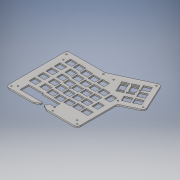
# Autodesk Inventor part: steelplate right
Saved by Autodesk Inventor 2016 (Build 200138000, 138)
## iProperties
Created: 2016-01-27
Part Number: steelplate right
Material: Generic
Document SubType Name: Sheet Metal
Designer: Fab Lab
Density: 1 g/cm^3
Sheet Metal Rule: Default
Appearance: Default
Author: Fab Lab
Autodesk Inventor part; units mm, degrees
ref_plane "YZ Plane" through (0, 0, 0) normal (1, 0, 0) x (0, 1, 0)
ref_plane "XZ Plane" through (0, 0, 0) normal (0, 1, 0) x (-1, 0, 0)
ref_plane "XY Plane" through (0, 0, 0) normal (0, 0, 1) x (1, 0, 0)
sketch "Sketch1" plane through (0, 0, 0) normal (0, 1, 0) x (-1, 0, 0)
  line L0 (-203.0862, 221.0628) -> (-258.5956, 221.0628)
  line L1 (-287.8818, 221.0628) -> (-350.173, 221.0628)
  line L2 (-342.06, 221.0628) -> (-350.173, 221.0628)
  line L3 (-277.102195, 211.948924) -> (-279.894095, 211.949068)
  line L4 (-269.4008, 215.9498) -> (-269.4008, 211.949)
  line L5 (-218.894185, 211.949) -> (-269.4008, 211.949)
  line L6 (-269.4008, 215.9498) -> (-267.9008, 215.9498)
  line L7 (-278.60199, 215.949801) -> (-277.10199, 215.949724)
  line L8 (-267.9008, 215.9498) -> (-258.5956, 221.0628)
  line L9 (-287.8818, 221.0628) -> (-278.5767, 215.9498)
  line L10 (-291.226534, 207.296649) -> (-279.894334, 207.296068)
  line L11 (-279.894095, 211.949068) -> (-279.894334, 207.296068)
  spline S0 degree 3 poles (-361.2149, 128.8298) (-358.7492, 129.9795) (-357.173, 132.4535) (-357.173, 135.174) knots 0 0 0 0 1 1 1 1
  line L12 (-361.2149, 128.8298) -> (-358.7492, 129.9795) construction
  line L13 (-358.7492, 129.9795) -> (-357.173, 132.4535) construction
  line L14 (-357.173, 132.4535) -> (-357.173, 135.174) construction
  spline S1 degree 3 poles (-280.219, 82.6328) (-281.241, 82.6328) (-282.2506, 82.409) (-283.1768, 81.9771) knots 0 0 0 0 1 1 1 1
  line L15 (-280.219, 82.6328) -> (-281.241, 82.6328) construction
  line L16 (-281.241, 82.6328) -> (-282.2506, 82.409) construction
  line L17 (-282.2506, 82.409) -> (-283.1768, 81.9771) construction
  line L18 (-357.172987, 214.0628) -> (-357.172987, 135.1741)
  line L19 (-196.0862, 89.6328) -> (-196.0862, 214.0628)
  line L20 (-398.011196, 103.949092) -> (-372.0468, 48.2678)
  line L21 (-362.7448, 44.8818) -> (-283.1768, 81.9771)
  line L22 (-280.219, 82.6328) -> (-203.0862, 82.6328)
  spline S2 degree 3 poles (-196.0862, 214.0628) (-196.0862, 215.9193) (-196.8237, 217.6997) (-198.1365, 219.0125) knots 0 0 0 0 1 1 1 1
  line L23 (-196.0862, 214.0628) -> (-196.0862, 215.9193) construction
  line L24 (-196.0862, 215.9193) -> (-196.8237, 217.6997) construction
  line L25 (-196.8237, 217.6997) -> (-198.1365, 219.0125) construction
  line L26 (-198.1365, 219.0125) -> (-198.1365, 219.0125) construction
  line L27 (-198.1365, 219.0125) -> (-199.4492, 220.3253) construction
  line L28 (-199.4492, 220.3253) -> (-201.2297, 221.0628) construction
  line L29 (-201.2297, 221.0628) -> (-203.0862, 221.0628) construction
  spline S3 degree 3 poles (-350.173, 221.0628) (-352.0295, 221.0628) (-353.81, 220.3253) (-355.1228, 219.0125) knots 0 0 0 0 1 1 1 1
  line L30 (-350.173, 221.0628) -> (-352.0295, 221.0628) construction
  line L31 (-352.0295, 221.0628) -> (-353.81, 220.3253) construction
  line L32 (-353.81, 220.3253) -> (-355.1228, 219.0125) construction
  line L33 (-355.1228, 219.0125) -> (-355.1228, 219.0125) construction
  line L34 (-355.1228, 219.0125) -> (-356.4355, 217.6997) construction
  line L35 (-356.4355, 217.6997) -> (-357.173, 215.9193) construction
  line L36 (-357.173, 215.9193) -> (-357.172987, 214.0628) construction
  line L37 (-361.2149, 128.8298) -> (-394.6251, 113.2517)
  spline S4 degree 3 poles (-203.0862, 82.6328) (-199.2202, 82.6328) (-196.0862, 85.7667) (-196.0862, 89.6327) knots 0 0 0 0 1 1 1 1
  line L38 (-203.0862, 82.6328) -> (-199.2202, 82.6328) construction
  line L39 (-199.2202, 82.6328) -> (-196.0862, 85.7667) construction
  line L40 (-196.0862, 85.7667) -> (-196.0862, 89.6327) construction
  spline S5 degree 3 poles (-372.0468, 48.2678) (-370.413, 44.7642) (-366.2485, 43.2483) (-362.7448, 44.8818) knots 0 0 0 0 1 1 1 1
  line L41 (-372.0468, 48.2678) -> (-370.413, 44.7642) construction
  line L42 (-370.413, 44.7642) -> (-366.2485, 43.2483) construction
  line L43 (-366.2485, 43.2483) -> (-362.7448, 44.8818) construction
  spline S6 degree 3 poles (-394.6251, 113.2517) (-396.3077, 112.4671) (-397.6098, 111.0463) (-398.2448, 109.3017) knots 0 0 0 0 1 1 1 1
  line L44 (-394.6251, 113.2517) -> (-396.3077, 112.4671) construction
  line L45 (-396.3077, 112.4671) -> (-397.6098, 111.0463) construction
  line L46 (-397.6098, 111.0463) -> (-398.2448, 109.3017) construction
  line L47 (-398.2448, 109.3017) -> (-398.2448, 109.3017) construction
  line L48 (-398.2448, 109.3017) -> (-398.8798, 107.5571) construction
  line L49 (-398.8798, 107.5571) -> (-398.7958, 105.6317) construction
  line L50 (-398.7958, 105.6317) -> (-398.011196, 103.949092) construction
  line L51 (-277.10199, 215.949724) -> (-277.102195, 211.948924)
  line L52 (-291.894992, 194.449787) -> (-291.894457, 206.045087)
  line L53 (-251.675985, 192.447826) -> (-218.895085, 192.446313)
  line L54 (-218.895085, 192.446313) -> (-218.894185, 211.949)
  line L55 (-251.675892, 194.447826) -> (-291.894992, 194.449683)
  line L56 (-251.675892, 194.447826) -> (-251.675985, 192.447826)
  line L57 (-227.2963, 171.6071) -> (-211.7963, 171.6071)
  line L58 (-211.7963, 171.6071) -> (-211.7963, 184.4071)
  line L59 (-211.7963, 184.4071) -> (-227.2963, 184.4071)
  line L60 (-227.2963, 184.4071) -> (-227.2963, 171.6071)
  line L61 (-251.0963, 171.6071) -> (-235.5963, 171.6071)
  line L62 (-235.5963, 171.6071) -> (-235.5963, 184.4071)
  line L63 (-235.5963, 184.4071) -> (-251.0963, 184.4071)
  line L64 (-251.0963, 184.4071) -> (-251.0963, 171.6071)
  line L65 (-227.2963, 152.5071) -> (-211.7963, 152.5071)
  line L66 (-211.7963, 152.5071) -> (-211.7963, 165.3071)
  line L67 (-211.7963, 165.3071) -> (-227.2963, 165.3071)
  line L68 (-227.2963, 165.3071) -> (-227.2963, 152.5071)
  line L69 (-251.0963, 152.5071) -> (-235.5963, 152.5071)
  line L70 (-235.5963, 152.5071) -> (-235.5963, 165.3071)
  line L71 (-235.5963, 165.3071) -> (-251.0963, 165.3071)
  line L72 (-251.0963, 165.3071) -> (-251.0963, 152.5071)
  line L73 (-227.2963, 133.5071) -> (-211.7963, 133.5071)
  line L74 (-211.7963, 133.5071) -> (-211.7963, 146.3071)
  line L75 (-211.7963, 146.3071) -> (-227.2963, 146.3071)
  line L76 (-227.2963, 146.3071) -> (-227.2963, 133.5071)
  line L77 (-251.0963, 133.5071) -> (-235.5963, 133.5071)
  line L78 (-235.5963, 133.5071) -> (-235.5963, 146.3071)
  line L79 (-235.5963, 146.3071) -> (-251.0963, 146.3071)
  line L80 (-251.0963, 146.3071) -> (-251.0963, 133.5071)
  line L81 (-227.2963, 114.5071) -> (-211.7963, 114.5071)
  line L82 (-211.7963, 114.5071) -> (-211.7963, 127.3071)
  line L83 (-211.7963, 127.3071) -> (-227.2963, 127.3071)
  line L84 (-227.2963, 127.3071) -> (-227.2963, 114.5071)
  line L85 (-251.0963, 114.5071) -> (-235.5963, 114.5071)
  line L86 (-235.5963, 114.5071) -> (-235.5963, 127.3071)
  line L87 (-235.5963, 127.3071) -> (-251.0963, 127.3071)
  line L88 (-251.0963, 127.3071) -> (-251.0963, 114.5071)
  line L89 (-270.0539, 174.7882) -> (-254.5539, 174.7882)
  line L90 (-254.5539, 174.7882) -> (-254.5539, 187.5882)
  line L91 (-254.5539, 187.5882) -> (-270.0539, 187.5882)
  line L92 (-270.0539, 187.5882) -> (-270.0539, 174.7882)
  line L93 (-270.0539, 155.6882) -> (-254.5539, 155.6882)
  line L94 (-254.5539, 155.6882) -> (-254.5539, 168.4882)
  line L95 (-254.5539, 168.4882) -> (-270.0539, 168.4882)
  line L96 (-270.0539, 168.4882) -> (-270.0539, 155.6882)
  line L97 (-270.0539, 136.6882) -> (-254.5539, 136.6882)
  line L98 (-254.5539, 136.6882) -> (-254.5539, 149.4882)
  line L99 (-254.5539, 149.4882) -> (-270.0539, 149.4882)
  line L100 (-270.0539, 149.4882) -> (-270.0539, 136.6882)
  line L101 (-270.0539, 117.6882) -> (-254.5539, 117.6882)
  line L102 (-254.5539, 117.6882) -> (-254.5539, 130.4882)
  line L103 (-254.5539, 130.4882) -> (-270.0539, 130.4882)
  line L104 (-270.0539, 130.4882) -> (-270.0539, 117.6882)
  line L105 (-270.0539, 98.5882) -> (-254.5539, 98.5882)
  line L106 (-254.5539, 98.5882) -> (-254.5539, 111.3882)
  line L107 (-254.5539, 111.3882) -> (-270.0539, 111.3882)
  line L108 (-270.0539, 111.3882) -> (-270.0539, 98.5882)
  line L109 (-289.1803, 176.3757) -> (-273.6803, 176.3757)
  line L110 (-273.6803, 176.3757) -> (-273.6803, 189.1757)
  line L111 (-273.6803, 189.1757) -> (-289.1803, 189.1757)
  line L112 (-289.1803, 189.1757) -> (-289.1803, 176.3757)
  line L113 (-289.1803, 157.2757) -> (-273.6803, 157.2757)
  line L114 (-273.6803, 157.2757) -> (-273.6803, 170.0757)
  line L115 (-273.6803, 170.0757) -> (-289.1803, 170.0757)
  line L116 (-289.1803, 170.0757) -> (-289.1803, 157.2757)
  line L117 (-289.1803, 138.2757) -> (-273.6803, 138.2757)
  line L118 (-273.6803, 138.2757) -> (-273.6803, 151.0757)
  line L119 (-273.6803, 151.0757) -> (-289.1803, 151.0757)
  line L120 (-289.1803, 151.0757) -> (-289.1803, 138.2757)
  line L121 (-289.1803, 119.2757) -> (-273.6803, 119.2757)
  line L122 (-273.6803, 119.2757) -> (-273.6803, 132.0757)
  line L123 (-273.6803, 132.0757) -> (-289.1803, 132.0757)
  line L124 (-289.1803, 132.0757) -> (-289.1803, 119.2757)
  line L125 (-289.1803, 100.1757) -> (-273.6803, 100.1757)
  line L126 (-273.6803, 100.1757) -> (-273.6803, 112.9757)
  line L127 (-273.6803, 112.9757) -> (-289.1803, 112.9757)
  line L128 (-289.1803, 112.9757) -> (-289.1803, 100.1757)
  line L129 (-308.1764, 174.8083) -> (-292.6764, 174.8083)
  line L130 (-292.6764, 174.8083) -> (-292.6764, 187.6083)
  line L131 (-292.6764, 187.6083) -> (-308.1764, 187.6083)
  line L132 (-308.1764, 187.6083) -> (-308.1764, 174.8083)
  line L133 (-308.1764, 155.7083) -> (-292.6764, 155.7083)
  line L134 (-292.6764, 155.7083) -> (-292.6764, 168.5083)
  line L135 (-292.6764, 168.5083) -> (-308.1764, 168.5083)
  line L136 (-308.1764, 168.5083) -> (-308.1764, 155.7083)
  line L137 (-308.1764, 136.7083) -> (-292.6764, 136.7083)
  line L138 (-292.6764, 136.7083) -> (-292.6764, 149.5083)
  line L139 (-292.6764, 149.5083) -> (-308.1764, 149.5083)
  line L140 (-308.1764, 149.5083) -> (-308.1764, 136.7083)
  line L141 (-308.1764, 117.7083) -> (-292.6764, 117.7083)
  line L142 (-292.6764, 117.7083) -> (-292.6764, 130.5083)
  line L143 (-292.6764, 130.5083) -> (-308.1764, 130.5083)
  line L144 (-308.1764, 130.5083) -> (-308.1764, 117.7083)
  line L145 (-308.1764, 98.6083) -> (-292.6764, 98.6083)
  line L146 (-292.6764, 98.6083) -> (-292.6764, 111.4083)
  line L147 (-292.6764, 111.4083) -> (-308.1764, 111.4083)
  line L148 (-308.1764, 111.4083) -> (-308.1764, 98.6083)
  line L149 (-327.2289, 173.5307) -> (-311.7289, 173.5307)
  line L150 (-311.7289, 173.5307) -> (-311.7289, 186.3307)
  line L151 (-311.7289, 186.3307) -> (-327.2289, 186.3307)
  line L152 (-327.2289, 186.3307) -> (-327.2289, 173.5307)
  line L153 (-327.2289, 154.4307) -> (-311.7289, 154.4307)
  line L154 (-311.7289, 154.4307) -> (-311.7289, 167.2307)
  line L155 (-311.7289, 167.2307) -> (-327.2289, 167.2307)
  line L156 (-327.2289, 167.2307) -> (-327.2289, 154.4307)
  line L157 (-327.2289, 135.4307) -> (-311.7289, 135.4307)
  line L158 (-311.7289, 135.4307) -> (-311.7289, 148.2307)
  line L159 (-311.7289, 148.2307) -> (-327.2289, 148.2307)
  line L160 (-327.2289, 148.2307) -> (-327.2289, 135.4307)
  line L161 (-327.2289, 116.4307) -> (-311.7289, 116.4307)
  line L162 (-311.7289, 116.4307) -> (-311.7289, 129.2307)
  line L163 (-311.7289, 129.2307) -> (-327.2289, 129.2307)
  line L164 (-327.2289, 129.2307) -> (-327.2289, 116.4307)
  line L165 (-346.3289, 173.5307) -> (-330.8289, 173.5307)
  line L166 (-330.8289, 173.5307) -> (-330.8289, 186.3307)
  line L167 (-330.8289, 186.3307) -> (-346.3289, 186.3307)
  line L168 (-346.3289, 186.3307) -> (-346.3289, 173.5307)
  line L169 (-251.0963, 95.4071) -> (-235.5963, 95.4071)
  line L170 (-235.5963, 95.4071) -> (-235.5963, 108.2071)
  line L171 (-235.5963, 108.2071) -> (-251.0963, 108.2071)
  line L172 (-251.0963, 108.2071) -> (-251.0963, 95.4071)
  line L173 (-231.9963, 95.4071) -> (-216.4963, 95.4071)
  line L174 (-216.4963, 95.4071) -> (-216.4963, 108.2071)
  line L175 (-216.4963, 108.2071) -> (-231.9963, 108.2071)
  line L176 (-231.9963, 108.2071) -> (-231.9963, 95.4071)
  line L177 (-332.7989, 147.8041) -> (-332.7989, 163.3041)
  line L178 (-332.7989, 163.3041) -> (-345.5989, 163.3041)
  line L179 (-345.5989, 163.3041) -> (-345.5989, 147.8041)
  line L180 (-345.5989, 147.8041) -> (-332.7989, 147.8041)
  line L181 (-332.7989, 119.2041) -> (-332.7989, 134.7041)
  line L182 (-332.7989, 134.7041) -> (-345.5989, 134.7041)
  line L183 (-345.5989, 134.7041) -> (-345.5989, 119.2041)
  line L184 (-345.5989, 119.2041) -> (-332.7989, 119.2041)
  line L185 (-354.9415, 118.8037) -> (-368.9892, 112.2531)
  line L186 (-368.9892, 112.2531) -> (-363.5797, 100.6523)
  line L187 (-363.5797, 100.6523) -> (-349.5319, 107.2029)
  line L188 (-349.5319, 107.2029) -> (-354.9415, 118.8037)
  line L189 (-372.2276, 110.778) -> (-386.2753, 104.2274)
  line L190 (-386.2753, 104.2274) -> (-380.8658, 92.6266)
  line L191 (-380.866146, 92.626439) -> (-366.81815, 99.17662)
  line L192 (-366.818, 99.1772) -> (-372.2276, 110.778)
  line L193 (-364.1137, 93.4918) -> (-378.1614, 86.9412)
  line L194 (-378.1614, 86.9412) -> (-372.7519, 75.3404)
  line L195 (-372.7519, 75.3404) -> (-358.7041, 81.891)
  line L196 (-358.7041, 81.891) -> (-364.1137, 93.4918)
  line L197 (-356.088, 76.2056) -> (-370.1357, 69.655)
  line L198 (-370.1357, 69.655) -> (-364.7262, 58.0542)
  line L199 (-364.7262, 58.0542) -> (-350.6784, 64.6048)
  line L200 (-350.678414, 64.604794) -> (-356.088, 76.2056)
  line L201 (-321.1491, 86.872) -> (-327.6997, 100.9198)
  line L202 (-327.6997, 100.9198) -> (-339.3004, 95.5103)
  line L203 (-339.3004, 95.5103) -> (-332.7499, 81.4625)
  line L204 (-332.7499, 81.4625) -> (-321.1491, 86.872)
  line L205 (-338.3471, 78.7581) -> (-344.8977, 92.8059)
  line L206 (-344.8977, 92.8059) -> (-356.4984, 87.3964)
  line L207 (-356.4984, 87.3964) -> (-349.9479, 73.3486)
  line L208 (-349.9479, 73.3486) -> (-338.347144, 78.758079)
  line L209 (-329.7631, 106.3199) -> (-328.3661, 103.3278)
  line L210 (-328.3676, 103.3271) -> (-341.032456, 97.430446)
  line L211 (-341.028, 97.4248) -> (-342.4225, 100.417)
  line L212 (-342.4225, 100.417) -> (-329.7631, 106.3199)
  line L213 (-319.6717, 84.6817) -> (-318.2772, 81.6895)
  line L214 (-318.2772, 81.6895) -> (-330.9366, 75.784)
  line L215 (-330.9366, 75.784) -> (-332.3336, 78.7762)
  line L216 (-332.3336, 78.7762) -> (-319.6717, 84.6817)
  line L217 (-346.8192, 68.3774) -> (-348.2162, 71.3695)
  line L218 (-348.2162, 71.3695) -> (-335.5543, 77.2725)
  line L219 (-335.5543, 77.2725) -> (-334.1599, 74.2804)
  line L220 (-334.158986, 74.280826) -> (-346.816481, 68.373958)
  line L221 (-356.9106, 90.0157) -> (-358.3051, 93.0078)
  line L222 (-358.3051, 93.0078) -> (-345.6457, 98.9133)
  line L223 (-345.6457, 98.9133) -> (-344.2487, 95.9212)
  line L224 (-344.2487, 95.9212) -> (-356.9106, 90.0157)
  spline S7 degree 3 poles (-358.587, 78.6034) (-358.587, 79.4451) (-357.9047, 80.1274) (-357.0631, 80.1274) knots 0 0 0 0 1 1 1 1
  line L225 (-358.587, 78.6034) -> (-358.587, 79.4451) construction
  line L226 (-358.587, 79.4451) -> (-357.9047, 80.1274) construction
  line L227 (-357.9047, 80.1274) -> (-357.0631, 80.1274) construction
  line L228 (-357.0631, 80.1274) -> (-357.0631, 80.1274) construction
  line L229 (-357.0631, 80.1274) -> (-356.2214, 80.1275) construction
  line L230 (-356.2214, 80.1275) -> (-355.5391, 79.4451) construction
  line L231 (-355.5391, 79.4451) -> (-355.539, 78.6035) construction
  line L232 (-355.539, 78.6035) -> (-355.539, 78.6035) construction
  line L233 (-355.539, 78.6035) -> (-355.539, 77.7618) construction
  line L234 (-355.539, 77.7618) -> (-356.2214, 77.0795) construction
  line L235 (-356.2214, 77.0795) -> (-357.063, 77.0794) construction
  spline S8 degree 3 poles (-357.063, 77.0794) (-357.063842, 77.0794) (-357.9047, 77.0794) (-358.587, 77.7618) (-358.587, 78.6034) knots 0 0 0 0 0.00000003 1 1 1 1
  line L236 (-357.063, 77.0794) -> (-357.063, 77.0794) construction
  line L237 (-357.063, 77.0794) -> (-357.9047, 77.0794) construction
  line L238 (-357.9047, 77.0794) -> (-358.587, 77.7618) construction
  line L239 (-358.587, 77.7618) -> (-358.587, 78.6034) construction
  spline S9 degree 3 poles (-352.8212, 122.774) (-352.8212, 123.6157) (-352.1389, 124.298) (-351.2973, 124.298) knots 0 0 0 0 1 1 1 1
  line L240 (-352.8212, 122.774) -> (-352.8212, 123.6157) construction
  line L241 (-352.8212, 123.6157) -> (-352.1389, 124.298) construction
  line L242 (-352.1389, 124.298) -> (-351.2973, 124.298) construction
  line L243 (-351.2973, 124.298) -> (-351.2973, 124.298) construction
  line L244 (-351.2973, 124.298) -> (-350.4556, 124.2981) construction
  line L245 (-350.4556, 124.2981) -> (-349.7733, 123.6157) construction
  line L246 (-349.7733, 123.6157) -> (-349.7732, 122.7741) construction
  line L247 (-349.7732, 122.7741) -> (-349.7732, 122.7741) construction
  line L248 (-349.7732, 122.7741) -> (-349.7732, 121.9324) construction
  line L249 (-349.7732, 121.9324) -> (-350.4556, 121.2501) construction
  line L250 (-350.4556, 121.2501) -> (-351.2972, 121.25) construction
  spline S10 degree 3 poles (-351.2972, 121.25) (-351.298042, 121.25) (-352.1389, 121.25) (-352.8212, 121.9324) (-352.8212, 122.774) knots 0 0 0 0 0.00000003 1 1 1 1
  line L251 (-351.2972, 121.25) -> (-351.2972, 121.25) construction
  line L252 (-351.2972, 121.25) -> (-352.1389, 121.25) construction
  line L253 (-352.1389, 121.25) -> (-352.8212, 121.9324) construction
  line L254 (-352.8212, 121.9324) -> (-352.8212, 122.774) construction
  spline S11 degree 3 poles (-307.0504, 86.6806) (-307.0504, 87.5223) (-306.3681, 88.2046) (-305.5265, 88.2046) knots 0 0 0 0 1 1 1 1
  line L255 (-307.0504, 86.6806) -> (-307.0504, 87.5223) construction
  line L256 (-307.0504, 87.5223) -> (-306.3681, 88.2046) construction
  line L257 (-306.3681, 88.2046) -> (-305.5265, 88.2046) construction
  line L258 (-305.5265, 88.2046) -> (-305.5265, 88.2046) construction
  line L259 (-305.5265, 88.2046) -> (-304.6848, 88.2047) construction
  line L260 (-304.6848, 88.2047) -> (-304.0025, 87.5223) construction
  line L261 (-304.0025, 87.5223) -> (-304.0024, 86.6807) construction
  line L262 (-304.0024, 86.6807) -> (-304.0024, 86.6807) construction
  line L263 (-304.0024, 86.6807) -> (-304.0024, 85.839) construction
  line L264 (-304.0024, 85.839) -> (-304.6848, 85.1567) construction
  line L265 (-304.6848, 85.1567) -> (-305.5264, 85.1566) construction
  spline S12 degree 3 poles (-305.5264, 85.1566) (-305.527242, 85.1566) (-306.3681, 85.1566) (-307.0504, 85.839) (-307.0504, 86.6806) knots 0 0 0 0 0.00000003 1 1 1 1
  line L266 (-305.5264, 85.1566) -> (-305.5264, 85.1566) construction
  line L267 (-305.5264, 85.1566) -> (-306.3681, 85.1566) construction
  line L268 (-306.3681, 85.1566) -> (-307.0504, 85.839) construction
  line L269 (-307.0504, 85.839) -> (-307.0504, 86.6806) construction
  spline S13 degree 3 poles (-210.7082, 104.3844) (-210.7082, 105.2261) (-210.0259, 105.9084) (-209.1843, 105.9084) knots 0 0 0 0 1 1 1 1
  line L270 (-210.7082, 104.3844) -> (-210.7082, 105.2261) construction
  line L271 (-210.7082, 105.2261) -> (-210.0259, 105.9084) construction
  line L272 (-210.0259, 105.9084) -> (-209.1843, 105.9084) construction
  line L273 (-209.1843, 105.9084) -> (-209.1843, 105.9084) construction
  line L274 (-209.1843, 105.9084) -> (-208.3426, 105.9085) construction
  line L275 (-208.3426, 105.9085) -> (-207.6603, 105.2261) construction
  line L276 (-207.6603, 105.2261) -> (-207.6602, 104.3845) construction
  line L277 (-207.6602, 104.3845) -> (-207.6602, 104.3845) construction
  line L278 (-207.6602, 104.3845) -> (-207.6602, 103.5428) construction
  line L279 (-207.6602, 103.5428) -> (-208.3426, 102.8605) construction
  line L280 (-208.3426, 102.8605) -> (-209.1842, 102.8604) construction
  spline S14 degree 3 poles (-209.1842, 102.8604) (-209.185042, 102.8604) (-210.0259, 102.8604) (-210.7082, 103.5428) (-210.7082, 104.3844) knots 0 0 0 0 0.00000003 1 1 1 1
  line L281 (-209.1842, 102.8604) -> (-209.1842, 102.8604) construction
  line L282 (-209.1842, 102.8604) -> (-210.0259, 102.8604) construction
  line L283 (-210.0259, 102.8604) -> (-210.7082, 103.5428) construction
  line L284 (-210.7082, 103.5428) -> (-210.7082, 104.3844) construction
  spline S15 degree 3 poles (-273.4462, 152.8476) (-273.4462, 153.6893) (-272.7639, 154.3716) (-271.9223, 154.3716) knots 0 0 0 0 1 1 1 1
  line L285 (-273.4462, 152.8476) -> (-273.4462, 153.6893) construction
  line L286 (-273.4462, 153.6893) -> (-272.7639, 154.3716) construction
  line L287 (-272.7639, 154.3716) -> (-271.9223, 154.3716) construction
  line L288 (-271.9223, 154.3716) -> (-271.9223, 154.3716) construction
  line L289 (-271.9223, 154.3716) -> (-271.0806, 154.3717) construction
  line L290 (-271.0806, 154.3717) -> (-270.3983, 153.6893) construction
  line L291 (-270.3983, 153.6893) -> (-270.3982, 152.8477) construction
  line L292 (-270.3982, 152.8477) -> (-270.3982, 152.8477) construction
  line L293 (-270.3982, 152.8477) -> (-270.3982, 152.006) construction
  line L294 (-270.3982, 152.006) -> (-271.0806, 151.3237) construction
  line L295 (-271.0806, 151.3237) -> (-271.9222, 151.3236) construction
  spline S16 degree 3 poles (-271.9222, 151.3236) (-271.923042, 151.3236) (-272.7639, 151.3236) (-273.4462, 152.006) (-273.4462, 152.8476) knots 0 0 0 0 0.00000003 1 1 1 1
  line L296 (-271.9222, 151.3236) -> (-271.9222, 151.3236) construction
  line L297 (-271.9222, 151.3236) -> (-272.7639, 151.3236) construction
  line L298 (-272.7639, 151.3236) -> (-273.4462, 152.006) construction
  line L299 (-273.4462, 152.006) -> (-273.4462, 152.8476) construction
  spline S17 degree 3 poles (-211.3432, 207.3052) (-211.3432, 208.1469) (-210.6609, 208.8292) (-209.8193, 208.8292) knots 0 0 0 0 1 1 1 1
  line L300 (-211.3432, 207.3052) -> (-211.3432, 208.1469) construction
  line L301 (-211.3432, 208.1469) -> (-210.6609, 208.8292) construction
  line L302 (-210.6609, 208.8292) -> (-209.8193, 208.8292) construction
  line L303 (-209.8193, 208.8292) -> (-209.8193, 208.8292) construction
  line L304 (-209.8193, 208.8292) -> (-208.9776, 208.8293) construction
  line L305 (-208.9776, 208.8293) -> (-208.2953, 208.1469) construction
  line L306 (-208.2953, 208.1469) -> (-208.2952, 207.3053) construction
  line L307 (-208.2952, 207.3053) -> (-208.2952, 207.3053) construction
  line L308 (-208.2952, 207.3053) -> (-208.2952, 206.4636) construction
  line L309 (-208.2952, 206.4636) -> (-208.9776, 205.7813) construction
  line L310 (-208.9776, 205.7813) -> (-209.8192, 205.7812) construction
  spline S18 degree 3 poles (-209.8192, 205.7812) (-209.820042, 205.7812) (-210.6609, 205.7812) (-211.3432, 206.4636) (-211.3432, 207.3052) knots 0 0 0 0 0.00000003 1 1 1 1
  line L311 (-209.8192, 205.7812) -> (-209.8192, 205.7812) construction
  line L312 (-209.8192, 205.7812) -> (-210.6609, 205.7812) construction
  line L313 (-210.6609, 205.7812) -> (-211.3432, 206.4636) construction
  line L314 (-211.3432, 206.4636) -> (-211.3432, 207.3052) construction
  spline S19 degree 3 poles (-294.2742, 207.3052) (-294.2742, 208.1469) (-293.5919, 208.8292) (-292.7503, 208.8292) knots 0 0 0 0 1 1 1 1
  line L315 (-294.2742, 207.3052) -> (-294.2742, 208.1469) construction
  line L316 (-294.2742, 208.1469) -> (-293.5919, 208.8292) construction
  line L317 (-293.5919, 208.8292) -> (-292.7503, 208.8292) construction
  line L318 (-292.7503, 208.8292) -> (-292.7503, 208.8292) construction
  line L319 (-292.7503, 208.8292) -> (-291.9086, 208.8293) construction
  line L320 (-291.9086, 208.8293) -> (-291.2263, 208.1469) construction
  line L321 (-291.2263, 208.1469) -> (-291.2262, 207.3053) construction
  line L322 (-291.2262, 207.3053) -> (-291.2262, 207.3053) construction
  line L323 (-291.2262, 207.3053) -> (-291.2262, 206.4636) construction
  line L324 (-291.2262, 206.4636) -> (-291.9086, 205.7813) construction
  line L325 (-291.9086, 205.7813) -> (-292.7502, 205.7812) construction
  spline S20 degree 3 poles (-292.7502, 205.7812) (-292.751042, 205.7812) (-293.5919, 205.7812) (-294.2742, 206.4636) (-294.2742, 207.3052) knots 0 0 0 0 0.00000003 1 1 1 1
  line L326 (-292.7502, 205.7812) -> (-292.7502, 205.7812) construction
  line L327 (-292.7502, 205.7812) -> (-293.5919, 205.7812) construction
  line L328 (-293.5919, 205.7812) -> (-294.2742, 206.4636) construction
  line L329 (-294.2742, 206.4636) -> (-294.2742, 207.3052) construction
  spline S21 degree 3 poles (-345.0742, 207.3052) (-345.0742, 208.1469) (-344.3919, 208.8292) (-343.5503, 208.8292) knots 0 0 0 0 1 1 1 1
  line L330 (-345.0742, 207.3052) -> (-345.0742, 208.1469) construction
  line L331 (-345.0742, 208.1469) -> (-344.3919, 208.8292) construction
  line L332 (-344.3919, 208.8292) -> (-343.5503, 208.8292) construction
  line L333 (-343.5503, 208.8292) -> (-343.5503, 208.8292) construction
  line L334 (-343.5503, 208.8292) -> (-342.7086, 208.8293) construction
  line L335 (-342.7086, 208.8293) -> (-342.0263, 208.1469) construction
  line L336 (-342.0263, 208.1469) -> (-342.0262, 207.3053) construction
  line L337 (-342.0262, 207.3053) -> (-342.0262, 207.3053) construction
  line L338 (-342.0262, 207.3053) -> (-342.0262, 206.4636) construction
  line L339 (-342.0262, 206.4636) -> (-342.7086, 205.7813) construction
  line L340 (-342.7086, 205.7813) -> (-343.5502, 205.7812) construction
  spline S22 degree 3 poles (-343.5502, 205.7812) (-343.551042, 205.7812) (-344.3919, 205.7812) (-345.0742, 206.4636) (-345.0742, 207.3052) knots 0 0 0 0 0.00000003 1 1 1 1
  line L341 (-343.5502, 205.7812) -> (-343.5502, 205.7812) construction
  line L342 (-343.5502, 205.7812) -> (-344.3919, 205.7812) construction
  line L343 (-344.3919, 205.7812) -> (-345.0742, 206.4636) construction
  line L344 (-345.0742, 206.4636) -> (-345.0742, 207.3052) construction
  spline S23 degree 3 poles (-298.9873, 216.627) (-298.9873, 217.4555) (-298.3158, 218.127) (-297.4873, 218.127) knots 0 0 0 0 1 1 1 1
  line L345 (-298.9873, 216.627) -> (-298.9873, 217.4555) construction
  line L346 (-298.9873, 217.4555) -> (-298.3158, 218.127) construction
  line L347 (-298.3158, 218.127) -> (-297.4873, 218.127) construction
  line L348 (-297.4873, 218.127) -> (-297.4873, 218.127) construction
  line L349 (-297.4873, 218.127) -> (-296.6589, 218.1271) construction
  line L350 (-296.6589, 218.1271) -> (-295.9874, 217.4555) construction
  line L351 (-295.9874, 217.4555) -> (-295.9873, 216.6271) construction
  line L352 (-295.9873, 216.6271) -> (-295.9873, 216.6271) construction
  line L353 (-295.9873, 216.6271) -> (-295.9873, 215.7986) construction
  line L354 (-295.9873, 215.7986) -> (-296.6589, 215.1271) construction
  line L355 (-296.6589, 215.1271) -> (-297.4873, 215.127) construction
  spline S24 degree 3 poles (-297.4873, 215.127) (-297.488129, 215.127) (-298.3158, 215.127) (-298.9873, 215.7986) (-298.9873, 216.627) knots 0 0 0 0 0.00000003 1 1 1 1
  line L356 (-297.4873, 215.127) -> (-297.4873, 215.127) construction
  line L357 (-297.4873, 215.127) -> (-298.3158, 215.127) construction
  line L358 (-298.3158, 215.127) -> (-298.9873, 215.7986) construction
  line L359 (-298.9873, 215.7986) -> (-298.9873, 216.627) construction
  spline S25 degree 3 poles (-352.4706, 214.8081) (-352.4706, 215.6365) (-351.799, 216.3081) (-350.9706, 216.3081) knots 0 0 0 0 1 1 1 1
  line L360 (-352.4706, 214.8081) -> (-352.4706, 215.6365) construction
  line L361 (-352.4706, 215.6365) -> (-351.799, 216.3081) construction
  line L362 (-351.799, 216.3081) -> (-350.9706, 216.3081) construction
  line L363 (-350.9706, 216.3081) -> (-350.9706, 216.3081) construction
  line L364 (-350.9706, 216.3081) -> (-350.1422, 216.3081) construction
  line L365 (-350.1422, 216.3081) -> (-349.4706, 215.6365) construction
  line L366 (-349.4706, 215.6365) -> (-349.4706, 214.8081) construction
  line L367 (-349.4706, 214.8081) -> (-349.4706, 214.8081) construction
  line L368 (-349.4706, 214.8081) -> (-349.4706, 213.9797) construction
  line L369 (-349.4706, 213.9797) -> (-350.1421, 213.3081) construction
  line L370 (-350.1421, 213.3081) -> (-350.9706, 213.3081) construction
  line L371 (-350.9706, 213.3081) -> (-350.9706, 213.3081) construction
  line L372 (-350.9706, 213.3081) -> (-351.799, 213.3081) construction
  line L373 (-351.799, 213.3081) -> (-352.4706, 213.9796) construction
  line L374 (-352.4706, 213.9796) -> (-352.4706, 214.8081) construction
  spline S26 degree 3 poles (-394.2125, 107.2724) (-394.2125, 108.1009) (-393.541, 108.7724) (-392.7125, 108.7724) knots 0 0 0 0 1 1 1 1
  line L375 (-394.2125, 107.2724) -> (-394.2125, 108.1009) construction
  line L376 (-394.2125, 108.1009) -> (-393.541, 108.7724) construction
  line L377 (-393.541, 108.7724) -> (-392.7125, 108.7724) construction
  line L378 (-392.7125, 108.7724) -> (-392.7125, 108.7724) construction
  line L379 (-392.7125, 108.7724) -> (-391.8841, 108.7724) construction
  line L380 (-391.8841, 108.7724) -> (-391.2125, 108.1009) construction
  line L381 (-391.2125, 108.1009) -> (-391.2125, 107.2724) construction
  line L382 (-391.2125, 107.2724) -> (-391.2125, 107.2724) construction
  line L383 (-391.2125, 107.2724) -> (-391.2125, 106.444) construction
  line L384 (-391.2125, 106.444) -> (-391.8841, 105.7724) construction
  line L385 (-391.8841, 105.7724) -> (-392.7125, 105.7724) construction
  line L386 (-392.7125, 105.7724) -> (-392.7125, 105.7724) construction
  line L387 (-392.7125, 105.7724) -> (-393.541, 105.7724) construction
  line L388 (-393.541, 105.7724) -> (-394.2125, 106.444) construction
  line L389 (-394.2125, 106.444) -> (-394.2125, 107.2724) construction
  spline S27 degree 3 poles (-367.6261, 50.2564) (-367.6261, 51.0848) (-366.9545, 51.7564) (-366.1261, 51.7564) knots 0 0 0 0 1 1 1 1
  line L390 (-367.6261, 50.2564) -> (-367.6261, 51.0848) construction
  line L391 (-367.6261, 51.0848) -> (-366.9545, 51.7564) construction
  line L392 (-366.9545, 51.7564) -> (-366.1261, 51.7564) construction
  line L393 (-366.1261, 51.7564) -> (-366.1261, 51.7564) construction
  line L394 (-366.1261, 51.7564) -> (-365.2977, 51.7564) construction
  line L395 (-365.2977, 51.7564) -> (-364.6261, 51.0848) construction
  line L396 (-364.6261, 51.0848) -> (-364.6261, 50.2564) construction
  line L397 (-364.6261, 50.2564) -> (-364.6261, 50.2564) construction
  line L398 (-364.6261, 50.2564) -> (-364.6261, 49.4279) construction
  line L399 (-364.6261, 49.4279) -> (-365.2977, 48.7564) construction
  line L400 (-365.2977, 48.7564) -> (-366.1261, 48.7564) construction
  line L401 (-366.1261, 48.7564) -> (-366.1261, 48.7564) construction
  line L402 (-366.1261, 48.7564) -> (-366.9545, 48.7564) construction
  line L403 (-366.9545, 48.7564) -> (-367.6261, 49.4279) construction
  line L404 (-367.6261, 49.4279) -> (-367.6261, 50.2563) construction
  spline S28 degree 3 poles (-284.3239, 87.087) (-284.3239, 87.9154) (-283.6523, 88.587) (-282.8239, 88.587) knots 0 0 0 0 1 1 1 1
  line L405 (-284.3239, 87.087) -> (-284.3239, 87.9154) construction
  line L406 (-284.3239, 87.9154) -> (-283.6523, 88.587) construction
  line L407 (-283.6523, 88.587) -> (-282.8239, 88.587) construction
  line L408 (-282.8239, 88.587) -> (-282.8239, 88.587) construction
  line L409 (-282.8239, 88.587) -> (-281.9955, 88.587) construction
  line L410 (-281.9955, 88.587) -> (-281.3239, 87.9154) construction
  line L411 (-281.3239, 87.9154) -> (-281.3239, 87.087) construction
  line L412 (-281.3239, 87.087) -> (-281.3239, 87.087) construction
  line L413 (-281.3239, 87.087) -> (-281.3239, 86.2585) construction
  line L414 (-281.3239, 86.2585) -> (-281.9955, 85.587) construction
  line L415 (-281.9955, 85.587) -> (-282.8239, 85.587) construction
  spline S29 degree 3 poles (-282.8239, 85.587) (-282.824728, 85.587) (-283.6523, 85.5869) (-284.3239, 86.2585) (-284.3239, 87.0869) knots 0 0 0 0 0.00000003 1 1 1 1
  line L416 (-282.8239, 85.587) -> (-282.8239, 85.587) construction
  line L417 (-282.8239, 85.587) -> (-283.6523, 85.5869) construction
  line L418 (-283.6523, 85.5869) -> (-284.3239, 86.2585) construction
  line L419 (-284.3239, 86.2585) -> (-284.3239, 87.0869) construction
  spline S30 degree 3 poles (-203.9179, 90.4933) (-203.9179, 91.3218) (-203.2463, 91.9933) (-202.4179, 91.9933) knots 0 0 0 0 1 1 1 1
  line L420 (-203.9179, 90.4933) -> (-203.9179, 91.3218) construction
  line L421 (-203.9179, 91.3218) -> (-203.2463, 91.9933) construction
  line L422 (-203.2463, 91.9933) -> (-202.4179, 91.9933) construction
  line L423 (-202.4179, 91.9933) -> (-202.4179, 91.9933) construction
  line L424 (-202.4179, 91.9933) -> (-201.5895, 91.9933) construction
  line L425 (-201.5895, 91.9933) -> (-200.9179, 91.3218) construction
  line L426 (-200.9179, 91.3218) -> (-200.9179, 90.4933) construction
  line L427 (-200.9179, 90.4933) -> (-200.9179, 90.4933) construction
  line L428 (-200.9179, 90.4933) -> (-200.9179, 89.6649) construction
  line L429 (-200.9179, 89.6649) -> (-201.5894, 88.9933) construction
  line L430 (-201.5894, 88.9933) -> (-202.4179, 88.9933) construction
  line L431 (-202.4179, 88.9933) -> (-202.4179, 88.9933) construction
  line L432 (-202.4179, 88.9933) -> (-203.2463, 88.9933) construction
  line L433 (-203.2463, 88.9933) -> (-203.9179, 89.6649) construction
  line L434 (-203.9179, 89.6649) -> (-203.9179, 90.4933) construction
  spline S31 degree 3 poles (-203.9179, 214.8081) (-203.9179, 215.6365) (-203.2463, 216.3081) (-202.4179, 216.3081) knots 0 0 0 0 1 1 1 1
  line L435 (-203.9179, 214.8081) -> (-203.9179, 215.6365) construction
  line L436 (-203.9179, 215.6365) -> (-203.2463, 216.3081) construction
  line L437 (-203.2463, 216.3081) -> (-202.4179, 216.3081) construction
  line L438 (-202.4179, 216.3081) -> (-202.4179, 216.3081) construction
  line L439 (-202.4179, 216.3081) -> (-201.5895, 216.3081) construction
  line L440 (-201.5895, 216.3081) -> (-200.9179, 215.6365) construction
  line L441 (-200.9179, 215.6365) -> (-200.9179, 214.8081) construction
  line L442 (-200.9179, 214.8081) -> (-200.9179, 214.8081) construction
  line L443 (-200.9179, 214.8081) -> (-200.9179, 213.9797) construction
  line L444 (-200.9179, 213.9797) -> (-201.5894, 213.3081) construction
  line L445 (-201.5894, 213.3081) -> (-202.4179, 213.3081) construction
  line L446 (-202.4179, 213.3081) -> (-202.4179, 213.3081) construction
  line L447 (-202.4179, 213.3081) -> (-203.2463, 213.3081) construction
  line L448 (-203.2463, 213.3081) -> (-203.9179, 213.9796) construction
  line L449 (-203.9179, 213.9796) -> (-203.9179, 214.8081) construction
  arc A0 (-291.226446, 207.296649) -> (-291.894457, 206.045087) centre (-292.750469, 207.306031) ccw
  circle A1 centre (-351.297077, 122.774) radius 1.524
  circle A2 centre (-357.062877, 78.6034) radius 1.524
  circle A3 centre (-366.126323, 50.2563) radius 1.5001
  circle A4 centre (-392.712377, 107.2724) radius 1.5
  circle A5 centre (-305.534178, 86.6727) radius 1.531919
  circle A6 centre (-282.8239, 87.0869) radius 1.5001
  circle A7 centre (-202.4179, 90.4933) radius 1.5
  circle A8 centre (-209.184077, 104.3844) radius 1.524
  circle A9 centre (-209.781506, 207.296) radius 1.533666
  circle A10 centre (-202.418023, 214.8081) radius 1.5
  circle A11 centre (-297.487177, 216.627) radius 1.5
  circle A12 centre (-350.970723, 214.8081) radius 1.5
  circle A13 centre (-343.559278, 207.296) radius 1.533199
  circle A14 centre (-271.9222, 152.847477) radius 1.524123
  circle A15 centre (-282.8239, 87.0869) radius 1.5001
  line L450 (-394.6251, 113.2517) -> (-394.625202, 113.25192)
  arc A16 (-394.625202, 113.25192) -> (-398.011196, 103.949092) centre (-391.666791, 106.907511) ccw
  arc A17 (-196.0862, 214.0628) -> (-203.0862, 221.0628) centre (-203.086362, 214.062638) ccw
  arc A18 (-350.173, 221.0628) -> (-357.172987, 214.0628) centre (-350.172987, 214.0628) ccw
  line L451 (-216.4963, 108.2071) -> (-231.9963, 108.2071)
  line L452 (-231.9963, 108.2071) -> (-231.9963, 95.4071)
  line L453 (-231.9963, 95.4071) -> (-216.4963, 95.4071)
  line L454 (-216.4963, 95.4071) -> (-216.4963, 108.2071)
  line L455 (-251.0963, 108.2071) -> (-235.5963, 108.2071)
  line L456 (-235.5963, 108.2071) -> (-235.5963, 95.4071)
  line L457 (-235.5963, 95.4071) -> (-251.0963, 95.4071)
  line L458 (-251.0963, 95.4071) -> (-251.0963, 108.2071)
  line L459 (-273.6803, 112.9757) -> (-289.1803, 112.9757)
  line L460 (-289.1803, 112.9757) -> (-289.1803, 100.1757)
  line L461 (-289.1803, 100.1757) -> (-273.6803, 100.1757)
  line L462 (-273.6803, 100.1757) -> (-273.6803, 112.9757)
  line L463 (-292.6764, 187.6083) -> (-308.1764, 187.6083)
  line L464 (-308.1764, 187.6083) -> (-308.1764, 174.8083)
  line L465 (-308.1764, 174.8083) -> (-292.6764, 174.8083)
  line L466 (-292.6764, 174.8083) -> (-292.6764, 187.6083)
  line L467 (-292.6764, 168.5083) -> (-308.1764, 168.5083)
  line L468 (-308.1764, 168.5083) -> (-308.1764, 155.7083)
  line L469 (-308.1764, 155.7083) -> (-292.6764, 155.7083)
  line L470 (-292.6764, 155.7083) -> (-292.6764, 168.5083)
  line L471 (-330.8289, 186.3307) -> (-346.3289, 186.3307)
  line L472 (-346.3289, 186.3307) -> (-346.3289, 173.5307)
  line L473 (-346.3289, 173.5307) -> (-330.8289, 173.5307)
  line L474 (-330.8289, 173.5307) -> (-330.8289, 186.3307)
  line L475 (-345.5989, 163.3041) -> (-332.7989, 163.3041)
  line L476 (-332.7989, 163.3041) -> (-332.7989, 147.8041)
  line L477 (-332.7989, 147.8041) -> (-345.5989, 147.8041)
  line L478 (-345.5989, 147.8041) -> (-345.5989, 163.3041)
  line L479 (-332.7989, 134.7041) -> (-345.5989, 134.7041)
  line L480 (-345.5989, 134.7041) -> (-345.5989, 119.2041)
  line L481 (-345.5989, 119.2041) -> (-332.7989, 119.2041)
  line L482 (-332.7989, 119.2041) -> (-332.7989, 134.7041)
  line L483 (-327.2289, 129.2307) -> (-311.7289, 129.2307)
  line L484 (-311.7289, 129.2307) -> (-311.7289, 116.4307)
  line L485 (-311.7289, 116.4307) -> (-327.2289, 116.4307)
  line L486 (-327.2289, 116.4307) -> (-327.2289, 129.2307)
  line L487 (-311.7289, 148.2307) -> (-327.2289, 148.2307)
  line L488 (-327.2289, 148.2307) -> (-327.2289, 135.4307)
  line L489 (-327.2289, 135.4307) -> (-311.7289, 135.4307)
  line L490 (-311.7289, 135.4307) -> (-311.7289, 148.2307)
  line L491 (-329.7631, 106.3199) -> (-328.3676, 103.3271)
  line L492 (-328.3676, 103.3271) -> (-341.027592, 97.423924)
  line L493 (-341.027592, 97.423924) -> (-342.423092, 100.416724)
  line L494 (-342.423092, 100.416724) -> (-329.7631, 106.3199)
  line L495 (-339.3004, 95.5103) -> (-332.7499, 81.4625)
  line L496 (-332.7499, 81.4625) -> (-321.149085, 86.871969)
  line L497 (-321.149085, 86.871969) -> (-327.699585, 100.919769)
  line L498 (-327.699585, 100.919769) -> (-339.3004, 95.5103)
  line L499 (-319.6717, 84.6817) -> (-332.3336, 78.7762)
  line L500 (-332.3336, 78.7762) -> (-330.937783, 75.783448)
  line L501 (-330.937783, 75.783448) -> (-318.275883, 81.688948)
  line L502 (-318.275883, 81.688948) -> (-319.6717, 84.6817)
  line L503 (-334.158986, 74.280826) -> (-335.5543, 77.2725)
  line L504 (-335.5543, 77.2725) -> (-348.215242, 71.367447)
  line L505 (-348.215242, 71.367447) -> (-346.819928, 68.375773)
  line L506 (-346.819928, 68.375773) -> (-334.158986, 74.280826)
  line L507 (-338.347144, 78.758079) -> (-344.8977, 92.8059)
  line L508 (-344.8977, 92.8059) -> (-356.498418, 87.396438)
  line L509 (-356.498418, 87.396438) -> (-349.947862, 73.348618)
  line L510 (-349.947862, 73.348618) -> (-338.347144, 78.758079)
  line L511 (-345.6457, 98.9133) -> (-344.2487, 95.9212)
  line L512 (-344.2487, 95.9212) -> (-356.908188, 90.010534)
  line L513 (-356.908188, 90.010534) -> (-358.305188, 93.002634)
  line L514 (-358.305188, 93.002634) -> (-345.6457, 98.9133)
  line L515 (-354.9415, 118.8037) -> (-349.5319, 107.2029)
  line L516 (-349.5319, 107.2029) -> (-363.579674, 100.652245)
  line L517 (-363.579674, 100.652245) -> (-368.989274, 112.253045)
  line L518 (-368.989274, 112.253045) -> (-354.9415, 118.8037)
  line L519 (-364.1137, 93.4918) -> (-358.7041, 81.891)
  line L520 (-358.7041, 81.891) -> (-372.751874, 75.340345)
  line L521 (-372.751874, 75.340345) -> (-378.161474, 86.941145)
  line L522 (-378.161474, 86.941145) -> (-364.1137, 93.4918)
  line L523 (-356.088, 76.2056) -> (-350.678414, 64.604794)
  line L524 (-350.678414, 64.604794) -> (-364.726182, 58.054162)
  line L525 (-364.726182, 58.054162) -> (-370.135768, 69.654968)
  line L526 (-370.135768, 69.654968) -> (-356.088, 76.2056)
  line L527 (-386.2753, 104.2274) -> (-380.866146, 92.626439)
  line L528 (-380.866146, 92.626439) -> (-366.817784, 99.176737)
  line L529 (-366.817784, 99.176737) -> (-372.226939, 110.777698)
  line L530 (-372.226939, 110.777698) -> (-386.2753, 104.2274)
  line L531 (-357.172987, 214.0628) -> (-357.173, 135.174)
  line L532 (-196.0862, 89.6327) -> (-196.0862, 214.0628)
  line L533 (-291.894457, 206.045087) -> (-291.894992, 194.449683)
  line L534 (-278.5767, 215.9498) -> (-277.10199, 215.949724)
  line L535 (-278.5767, 215.9498) -> (-287.8818, 221.0628)
  point P0 (0, 0)
extrude "Plate1" add sketch "Sketch1" along normal blind 3.048 contours A17 S2 L19 S4 L22 S1 L21 S5 L20 A16 S6 L37 S0 L18 A18 S3 L1 L9 L7 L51 L3 L11 L10 A0 S19 S20 L52 L55 L56 L53 L54 L5 L4 L6 L8 L0 | L217 L218 L504 | L221 L222 L514 | S17 A9 S18
equation "\"BendRadius\" = Thickness"
equation "\"BendReliefWidth\" = Thickness"
equation "\"BendReliefDepth\" = 0.5 * Thickness"
equation "\"CornerReliefSize\" = 4 * Thickness"
equation "\"MinimumRemnant\" = 2 * Thickness"
equation "\"TransitionRadius\" = BendRadius"
equation "\"JacobiRadiusSize\" = BendRadius"
equation "\"GapSize\" = Thickness"
equation "\"d0\" = BendRadius"
equation "\"Thickness\" = 3.048"
body "Solid1"
